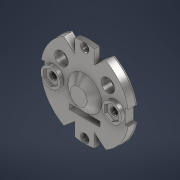
# Autodesk Inventor part: 18102021-002-02
Saved by Autodesk Inventor 2021 (Build 250183000, 183)
## iProperties
Created: 2021-10-15
Part Number: 18102021-002-02
Material: Stainless Steel
Document SubType Name: Modeling
Designer: DuctopwH
Density: 8 g/cm^3
Appearance: Semi-Polished
Author: DuctopwH
Autodesk Inventor part; units mm, degrees
ref_plane "YZ Plane" through (0, 0, 0) normal (1, 0, 0) x (0, 1, 0)
ref_plane "XZ Plane" through (0, 0, 0) normal (0, 1, 0) x (-1, 0, 0)
ref_plane "XY Plane" through (0, 0, 0) normal (0, 0, 1) x (1, 0, 0)
sketch "Sketch1" plane through (0, 0, 0) normal (0, 0, 1) x (1, 0, 0)
  circle A0 centre (0, 0) radius 18
  line L0 (0, 0) -> (0, 18) construction
  line L1 (4, 17.5499) -> (4, 11.9999)
  line L2 (4, 11.9999) -> (8.5659, 15.8312)
  line L3 (0, 0) -> (18, 0) construction
  line L4 (-4, 17.5499) -> (-4, 11.9999)
  line L5 (-4, 11.9999) -> (-8.5659, 15.8312)
  line L6 (4, -17.5499) -> (4, -11.9999)
  line L7 (4, -11.9999) -> (8.5659, -15.8312)
  line L8 (-4, -11.9999) -> (-8.5659, -15.8312)
  line L9 (-4, -17.5499) -> (-4, -11.9999)
  dimension "d1" = 50
  dimension "d2" = 36
  dimension "d3" = 5.55
  dimension "d4" = 8
  constraints: 20 end point, 9 symmetric about line, 4 point on circle, 2 vertical, 1 centre point, 1 coincident, 1 horizontal
  measures "d1" angle of L2 L1
  measures "d2" diameter of A0
  measures "d3" distance of L5.start L4.start
  measures "d4" distance between parallel lines of L1 L4
extrude "Extrusion1" add sketch "Sketch1" along normal blind 3.5
sketch "Sketch2" plane through (0, 0, 0) normal (0, 1, 0) x (-1, 0, 0)
  line L0 (0, 0) -> (0, 6)
  line L1 (0, 6) -> (-3.5, 6)
  line L2 (-3.5, 6) -> (-6.875, 3.5)
  line L3 (8.5659, 3.5) -> (-18, 3.5) projected
  line L4 (8.5659, 0) -> (8.5659, 0) projected
  line L5 (-6.875, 3.5) -> (0, 3.5)
  line L6 (-8.5659, 3.5) -> (-4, 3.5) projected
  point P0 (-18, 0)
  point P1 (18, 0)
  dimension "d7" = 3.5
  dimension "d8" = 6
  dimension "d9" = 13.75
  constraints: 8 end point, 2 point on line, 1 collinear, 1 perpendicular, 1 vertical, 1 other
  measures "d7" distance from line of L0 L1.end
  measures "d8" distance of the line from the sketch origin of L1
  measures "d9" diameter of L2.end L0
revolve "Revolution1" add sketch "Sketch2" angle 360 about axis through (0, 0, 0) along (0, 0, 1)
sketch "Sketch6" plane through (0, 0, 0) normal (1, 0, 0) x (0, 1, 0)
  circle A0 centre (-18, 0.2) radius 0.2
  line L0 (18, 0) -> (-18, 0) projected
  line L1 (-18, 0) -> (-18, 3.5) projected
  line L2 (0, 0) -> (0, 9.8131)
  point P0 (-18, 0.4)
  dimension "d28" = 0.4
  constraints: 2 end point, 1 centre point, 1 point on line, 1 tangent, 1 vertical
  measures "d28" diameter of A0
revolve "Revolution2" add sketch "Sketch6" angle 360 about axis through (0, 0, 0) along (0, 0, 1) picked at (-18.0623, 0.1764) contours A0 L1
sketch "Sketch7" plane through (0, 0, 3.5) normal (0, 0, 1) x (1, 0, 0)
  line L0 (4, 17.5499) -> (4, 11.9999) projected
  line L1 (4, 11.9999) -> (8.5659, 15.8312) projected
  line L2 (-4, 17.5499) -> (-4, 11.9999) projected
  line L3 (-4, 11.9999) -> (-8.5659, 15.8312) projected
  line L4 (-4, -11.9999) -> (-8.5659, -15.8312) projected
  line L5 (-4, -17.5499) -> (-4, -11.9999) projected
  line L6 (4, -17.5499) -> (4, -11.9999) projected
  line L7 (4, -11.9999) -> (8.5659, -15.8312) projected
  line L8 (4, -17.5499) -> (4, -18.3914)
  line L9 (8.5659, -15.8312) -> (9.2402, -16.397)
  line L10 (0, 0) -> (0, -19.1276)
  line L11 (0, 0) -> (-12.703, 0)
  circle A0 centre (0, 0) radius 18.8214
  line L12 (-4, -17.5499) -> (-4, -18.3914)
  line L13 (-8.5659, -15.8312) -> (-9.2402, -16.397)
  line L14 (4, 17.5499) -> (4, 18.3914)
  line L15 (8.5659, 15.8312) -> (9.2402, 16.397)
  line L16 (-4, 17.5499) -> (-4, 18.3914)
  line L17 (-8.5659, 15.8312) -> (-9.2402, 16.397)
  constraints: 20 end point, 6 symmetric about line, 2 point on circle, 2 vertical, 1 centre point, 1 coincident, 1 collinear, 1 horizontal
extrude "Extrusion5" cut sketch "Sketch7" against normal through all contours L14 A0 L15 L1 L0 | L16 L2 L3 L17 A0 | A0 L8 L6 L7 L9 | L13 L4 L5 L12 A0
sketch "Sketch4" plane through (0, 0, 3.5) normal (0, 0, 1) x (1, 0, 0)
  line L0 (0, 0) -> (0, -18)
  arc A0 (-8.5659, 15.8312) -> (-8.5659, -15.8312) centre (0, 0) ccw projected
  line L1 (0, -8.925) -> (-6.25, -8.925)
  line L2 (-6.25, -8.925) -> (-6.25, -6.875)
  line L3 (-6.25, -6.875) -> (0, -6.875)
  circle A1 centre (0, 0) radius 6.875 projected
  line L4 (0, -8.925) -> (6.25, -8.925)
  line L5 (6.25, -8.925) -> (6.25, -6.875)
  line L6 (6.25, -6.875) -> (0, -6.875)
  point P0 (-4, -17.5499)
  point P1 (4, -17.5499)
  dimension "d12" = 2.05
  dimension "d13" = 12.5
  constraints: 14 end point, 2 horizontal, 2 point on line, 2 symmetric about line, 1 perpendicular, 1 point on circle, 1 vertical, 1 vertical alignment, 1 other
  measures "d12" distance of L1.end L2.end
  measures "d13" distance between parallel lines of L5 L2
extrude "Extrusion2" cut sketch "Sketch4" against normal through all contours L6 L5 L4 L0 | L0 L1 L2 L3
sketch "Sketch3" plane through (0, 0, 0) normal (0, 0, -1) x (-1, 0, 0)
  line L0 (8.5659, -15.8312) -> (4, -11.9999) projected
  line L1 (8.5659, -15.8312) -> (4, -11.9999)
  line L2 (4, -11.9999) -> (8, -11.9999)
  line L3 (8, -11.9999) -> (8, -3.9)
  line L4 (8, -3.9) -> (-1.347, -3.9)
  line L5 (0, 0) -> (0, -22.6953) construction
  line L6 (8.5659, -15.8312) -> (9.347, -21.3508)
  line L7 (9.347, -21.3508) -> (0, -21.3508)
  line L8 (4, 11.9999) -> (8.5659, 15.8312) projected
  line L9 (8.5659, 15.8312) -> (4, 11.9999)
  line L10 (4, 11.9999) -> (-4, 11.9999)
  line L11 (-8.5659, 15.8312) -> (-4, 11.9999) projected
  line L12 (-4, 11.9999) -> (-8.5659, 15.8312)
  line L13 (-8.5659, 15.8312) -> (-8.5659, 22.0204)
  line L14 (-8.5659, 22.0204) -> (9.347, 21.5839)
  line L15 (9.347, 21.5839) -> (8.5659, 15.8312)
  line L16 (-8.5659, -15.8312) -> (-4, -11.9999)
  line L17 (-4, -11.9999) -> (-8, -11.9999)
  line L18 (-8, -11.9999) -> (-8, -3.9)
  line L19 (-8, -3.9) -> (-1.347, -3.9)
  line L20 (-8.5659, -15.8312) -> (-9.347, -21.3508)
  line L21 (-9.347, -21.3508) -> (0, -21.3508)
  line L22 (6.25, -8.925) -> (6.25, -6.875) projected
  line L23 (6.25, -7.9) -> (0, -7.9) construction
  line L24 (6.25, -7.9) -> (6.25, -5.4)
  line L25 (6.25, -5.4) -> (6.25, -3.9)
  dimension "d11" = 16
  dimension "d16" = 2.5
  dimension "d17" = 1.5
  constraints: 44 end point, 5 point on line, 5 symmetric about line, 4 horizontal, 3 collinear, 3 perpendicular, 1 midpoint, 1 vertical
  measures "d11" distance between parallel lines of L18 L3
  measures "d16" distance from line of L24.end L23
  measures "d17" distance of L24.end L25.end
extrude "Extrusion3" cut sketch "Sketch3" against normal blind 1.5
sketch "Sketch5" plane through (0, 0, 0) normal (1, 0, 0) x (0, 1, 0)
  line L0 (-6.875, 1.5) -> (-8.925, 1.5) projected
  line L1 (-6.875, 1.5) -> (-6.875, -2.7432)
  line L2 (-11.9999, 1.5) -> (-3.9, 1.5) projected
  line L3 (-5.45, 1.5) -> (-5.7054, -2.1568)
  line L4 (-7.95, 1.5) -> (-7.95, -5) construction
  circle A0 centre (-7.95, -2) radius 1.25
  circle A1 centre (-7.95, -5) radius 2.5
  circle A2 centre (-7.95, -2) radius 2.25
  line L5 (-10.45, 1.5) -> (-10.1945, -2.1568)
  line L6 (-6.875, 3.5) -> (-8.925, 3.5) projected
  line L7 (-8.925, 3.5) -> (-8.925, 1.5) projected
  line L8 (-8.925, 1.5) -> (-8.925, -1.2178)
  line L9 (-8.925, 0.0278) -> (-8.925, -1.2178)
  line L10 (-5.45, 1.5) -> (-5.45, 0) construction
  line L11 (-11.9999, 0) -> (-3.9, 0) projected
  point P0 (0, 0)
  point P1 (-9.0249, -0.0234)
  point P2 (-6.875, -1.3621)
  point P3 (-6.9273, -2.7187)
  point P4 (-6.115, -3.3021)
  point P5 (-9.7849, -3.3021)
  point P6 (-8.9727, -2.7188)
  point P7 (-6.875, -2.6379)
  point P8 (-6.875, -2.7429)
  dimension "d21" = 2.5
  dimension "d20" = 5
  dimension "d22" = 4.5
  dimension "d23" = 5
  dimension "d24" = 5.5
  dimension "d25" = 3
  constraints: 14 end point, 4 point on line, 3 point on circle, 3 vertical, 2 centre point, 2 coincident, 2 collinear, 2 symmetric about line, 1 midpoint, 1 tangent, 3 other
  measures "d20" distance of L5.start L3.start
  measures "d22" diameter of A2
  measures "d23" diameter of A1
  measures "d24" distance from line of L6 point (-7.95, -2)
  measures "d25" distance of L4.end point (-7.95, -2)
extrude "Extrusion4" add sketch "Sketch5" along normal mid plane 12.5 contours L2 L3 L11 L1 | L8 A2 L11 L5 L2 | L11 L3 A2 L1 | L8 L11 A2 | A2 A1 L1 A0 | L11 A2 L5 | L11 L8 A0 A1 A2 | L1 A1 A0 picked at (-8.956, 0.0031) picked at (-6.8805, -2.682)
sketch "Sketch9" plane through (0, 0, 3.5) normal (0, 0, 1) x (1, 0, 0)
  line L0 (0, 0) -> (0, 19.9091)
  line L1 (0, 0) -> (-25.5758, 0)
  line L2 (-20.3636, 0) -> (-20.3636, 3)
  line L3 (-20.3636, 3) -> (-16.5, 3)
  line L4 (-16.5, 3) -> (-16.5, 0)
  line L5 (-20.3636, 0) -> (-20.3636, -3)
  line L6 (-16.5, -3) -> (-16.5, 0)
  line L7 (-20.3636, -3) -> (-16.5, -3)
  line L8 (20.3636, 0) -> (20.3636, 3)
  line L9 (20.3636, 3) -> (16.5, 3)
  line L10 (16.5, 3) -> (16.5, 0)
  line L11 (20.3636, 0) -> (20.3636, -3)
  line L12 (16.5, -3) -> (16.5, 0)
  line L13 (20.3636, -3) -> (16.5, -3)
  dimension "d34" = 6
  dimension "d35" = 33
  constraints: 28 end point, 8 symmetric about line, 2 perpendicular, 2 point on line, 2 vertical, 1 horizontal, 1 parallel
  measures "d34" distance between parallel lines of L7 L3
  measures "d35" distance between parallel lines of L10 L4
extrude "Extrusion6" cut sketch "Sketch9" against normal through all
sketch "Sketch10" plane through (0, 0, 3.5) normal (0, 0, 1) x (1, 0, 0)
  circle A0 centre (-12.5, 0) radius 4
  line L0 (-12.5, 3.2505) -> (-9.685, 1.6252)
  line L1 (-9.685, 1.6252) -> (-9.685, -1.6252)
  line L2 (-9.685, -1.6252) -> (-12.5, -3.2505)
  line L3 (-12.5, -3.2505) -> (-15.315, -1.6252)
  line L4 (-15.315, -1.6252) -> (-15.315, 1.6252)
  line L5 (-15.315, 1.6252) -> (-12.5, 3.2505)
  line L6 (-12.5, 0) -> (-12.5, 3.2505)
  line L7 (-16.5, 3) -> (-16.5, -3) projected
  line L8 (0, 0) -> (0, 18.074)
  circle A1 centre (12.5, 0) radius 4
  line L9 (12.5, 3.2505) -> (9.685, 1.6252)
  line L10 (9.685, 1.6252) -> (9.685, -1.6252)
  line L11 (9.685, -1.6252) -> (12.5, -3.2505)
  line L12 (12.5, -3.2505) -> (15.315, -1.6252)
  line L13 (15.315, -1.6252) -> (15.315, 1.6252)
  line L14 (15.315, 1.6252) -> (12.5, 3.2505)
  line L15 (12.5, 0) -> (12.5, 3.2505)
  dimension "d38" = 8
  dimension "d42" = 5.63
  constraints: 30 end point, 8 symmetric about line, 2 centre point, 2 coincident, 2 vertical, 1 horizontal alignment, 1 tangent, 14 other
  measures "d38" diameter of A0
  measures "d42" distance between parallel lines of L1 L4
extrude "Extrusion7" add sketch "Sketch10" along normal blind 5 from surface at -3.5
sketch "Sketch11" plane through (0, 0, 3.5) normal (0, 0, 1) x (1, 0, 0)
  circle A0 centre (-12.5, 0) radius 4 projected
  circle A1 centre (-12.5, 0) radius 1.25
  circle A2 centre (0, 16) radius 1.5
  circle A3 centre (-9.5, 7.5) radius 2.75
  line L0 (0, 0) -> (0, 18) construction
  arc A4 (4, 17.5499) -> (-4, 17.5499) centre (0, 0) ccw projected
  line L1 (0, 0) -> (6.926, 0) construction
  circle A5 centre (0, -16) radius 1.5
  circle A6 centre (12.5, 0) radius 1.25
  circle A7 centre (9.5, 7.5) radius 2.75
  point P0 (-16.5, 0)
  dimension "d43" = 2.5
  dimension "d44" = 3
  dimension "d45" = 5.5
  dimension "d46" = 7.5
  dimension "d47" = 19
  dimension "d48" = 32
  constraints: 6 centre point, 4 end point, 3 symmetric about line, 1 coincident, 1 horizontal, 1 horizontal alignment, 1 point on circle, 1 point on line, 1 vertical, 3 other
  measures "d43" diameter of A1
  measures "d44" diameter of A2
  measures "d45" diameter of A3
  measures "d46" vertical distance of A6.centre A7.centre
  measures "d47" distance of A3.centre A7.centre
  measures "d48" distance of A2.centre A5.centre
extrude "Extrusion8" cut sketch "Sketch11" against normal through all contours A1 | A2 | A3 | A5 | A6 | A7
sketch "Sketch12" plane through (0, 0, 0) normal (0, 0, -1) x (-1, 0, 0)
  circle A0 centre (0, 0) radius 2
  dimension "d54" = 4
  constraints: 1 centre point, 1 coincident
  measures "d54" diameter of A0
extrude "Extrusion9" cut sketch "Sketch12" against normal blind 3.5
sketch "Sketch13" plane through (0, 0, 3.5) normal (0, 0, 1) x (1, 0, 0)
  circle A0 centre (12.5, 0) radius 1.25 projected
  line L0 (12.5, 3.2505) -> (9.685, 1.6252) projected
  line L1 (9.685, 1.6252) -> (9.685, -1.6252) projected
  line L2 (9.685, -1.6252) -> (12.5, -3.2505) projected
  line L3 (12.5, -3.2505) -> (15.315, -1.6252) projected
  line L4 (15.315, -1.6252) -> (15.315, 1.6252) projected
  line L5 (15.315, 1.6252) -> (12.5, 3.2505) projected
  circle A1 centre (-12.5, 0) radius 1.25 projected
  line L6 (-12.5, 3.2505) -> (-15.315, 1.6252) projected
  line L7 (-15.315, 1.6252) -> (-15.315, -1.6252) projected
  line L8 (-15.315, -1.6252) -> (-12.5, -3.2505) projected
  line L9 (-12.5, -3.2505) -> (-9.685, -1.6252) projected
  line L10 (-9.685, -1.6252) -> (-9.685, 1.6252) projected
  line L11 (-9.685, 1.6252) -> (-12.5, 3.2505) projected
  point P0 (0, 0)
extrude "Extrusion10" add sketch "Sketch13" along normal blind 0.5
chamfer "Chamfer2" distance 0.3 angle 45 6 edges at (11.25, 0, 4) (-13.75, 0, 4) (-1.5, -16, 3.5) (-1.5, 16, 3.5) (-13.75, 0, 0) (11.25, 0, 0)
body "Solid1"
